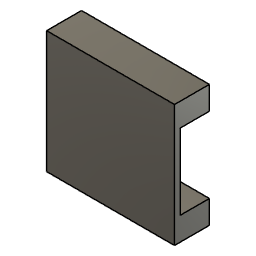
磁铁测试底座 (Autodesk Fusion 360 design; units mm, degrees)
Autodesk Fusion 360 part; units mm, degrees
note: some values were not read from the file. Chosen so that the rebuilt part matches the saved one: which bodies a step acts on.
sketch "草图1" plane through (0, 0, 0) normal (0, 1, 0) x (1, 0, 0)
  line L0 (0, 0) -> (22, 0)
  line L1 (22, 0) -> (22, -6)
  line L2 (22, -6) -> (0, -6)
  line L3 (0, -6) -> (0, 0)
  line L4 (1, -5) -> (21, -5)
  line L5 (21, -5) -> (21, 0)
  line L6 (21, 0) -> (1, 0)
  line L7 (1, 0) -> (1, -5)
  dimension "d1" = 22
  dimension "d2" = 6
  dimension "d3" = 1
  dimension "d4" = 1
  dimension "d5" = 1
  constraint horizontal L0
  constraint vertical L1
  constraint horizontal L2
  constraint vertical L3
  constraint coincident L0.start L3.end
  constraint horizontal L4
  constraint vertical L5
  constraint horizontal L6
  constraint vertical L7
  constraint coincident L0 L5.end
  measures "d1" distance of L0.start L0.end
  measures "d2" distance of L0.start L2.end
  measures "d3" distance of L2 L4
  measures "d4" distance of L3 L7
  measures "d5" distance of L1 L5
extrude "拉伸1" add sketch "草图1" along normal blind 21 contours L0 L1 L2 L3 L4 L5 L7 makes body 1
extrude "拉伸2" add sketch "草图1" along normal blind 1 separate body contours L0 L4 L5 L6 L7 makes body 2
sketch "草图2" plane through (0, 0, 5) normal (0, 0, -1) x (-1, 0, 0)
  line L0 (-21, 0) -> (-1, 0)
  line L1 (-1, 0) -> (-1, 21)
  line L2 (-1, 21) -> (-21, 21)
  line L3 (-21, 21) -> (-21, 0)
  line L4 (-1, 20) -> (-21, 20)
  line L5 (-21, 20) -> (-21, 21)
  line L6 (-21, 21) -> (-1, 21)
  line L7 (-1, 21) -> (-1, 20)
  line L8 (-21, 20) -> (-21, 18)
  line L9 (-1, 1) -> (-1, 3)
  line L10 (-22, 18) -> (0, 18)
  line L11 (0, 18) -> (0, 3)
  line L12 (0, 3) -> (-22, 3)
  line L13 (-22, 3) -> (-22, 18)
  dimension "d10" = 1
  constraint horizontal L4
  constraint vertical L5
  constraint horizontal L6
  constraint vertical L7
  constraint coincident L2.end L3.start
  constraint coincident L1 L4.start
  constraint coincident L3 L8.end
  constraint perpendicular L4 L8
  constraint coincident L1 L9.start
  constraint coincident L1 L9.end
  constraint horizontal L10
  constraint vertical L11
  constraint horizontal L12
  constraint vertical L13
  measures "d10" distance of L4 L6
extrude "拉伸3" add sketch "草图2" along normal blind 5 contours L1 L2 L3 L4 L5 L6 L7 bodies 1
sketch "草图3" plane through (0, 0, 5) normal (0, 0, -1) x (-1, 0, 0)
  line L0 (-1, 20) -> (-21, 20)
  line L1 (-21, 20) -> (-21, 0)
  line L2 (-21, 0) -> (-1, 0)
  line L3 (-1, 0) -> (-1, 20)
  line L4 (-1, 1) -> (-1, 3)
  line L5 (-1, 20) -> (-1, 18)
  line L6 (-1, 3) -> (0, 3)
  line L7 (0, 3) -> (0, 18)
  line L8 (0, 18) -> (-1, 18)
  line L9 (-1, 18) -> (-1, 3)
  line L10 (-21, 3) -> (-22, 3)
  line L11 (-22, 3) -> (-22, 18)
  line L12 (-22, 18) -> (-21, 18)
  line L13 (-21, 18) -> (-21, 3)
  line L14 (0, 10.5) -> (-11, 10.5) construction
  line L15 (-11, 10.5) -> (-11, 10) construction
  line L16 (-11, 10) -> (-15, 10)
  line L17 (-15, 10) -> (-17.5, 9.5)
  line L18 (-17.5, 9.5) -> (-15, 9)
  line L19 (-15, 9) -> (-7.5, 9)
  line L20 (-7.5, 9) -> (-5, 9.5)
  line L21 (-5, 9.5) -> (-7.5, 10)
  line L22 (-7.5, 10) -> (-11, 10)
  line L23 (-22, 10) -> (0, 10)
  dimension "d13" = 2
  dimension "d14" = 2
  constraint coincident L3 L4.start
  constraint coincident L0.start L3.end
  constraint coincident L3 L5.end
  constraint horizontal L6
  constraint vertical L7
  constraint horizontal L8
  constraint vertical L9
  constraint horizontal L10
  constraint vertical L11
  constraint horizontal L12
  constraint vertical L13
  constraint coincident L1 L10.start
  constraint midpoint L7 L14.start
  constraint perpendicular L11 L14
  constraint perpendicular L14 L15
  constraint perpendicular L15 L16
  constraint parallel L16 L19
  constraint parallel L17 L20
  constraint parallel L18 L21
  constraint perpendicular L15 L22
  constraint coincident L11 L23.start
  constraint coincident L7 L23.end
  constraint perpendicular L7 L23
  measures "d13" distance of L4.start L4.end
  measures "d14" distance of L0.start L5.end
extrude "拉伸5" cut sketch "草图3" against normal blind 1 contours L16 L17 L18 L19 L20 L21 L22 L23 bodies 1
pattern_linear "R-阵列1" count 9 spacing 1 along (0, -1, 0) of "拉伸5"
extrude "拉伸1'" add sketch "草图3" against normal blind 1 separate body contours L16 L17 L18 L19 L20 L21 L22 L23 makes body 3 in component "Component'"
pattern_linear "R-阵列1'" count 9 spacing 1 along (0, -1, 0) of "拉伸1'" makes body 4 makes body 5 makes body 6 makes body 7 makes body 8 makes body 9 makes body 10 makes body 11 in component "Component'"
split "分割1" by curves path "草图3" along L23 bodies 1 makes body 12 at (1.6667, 4.8333, 6)
sketch "草图4" plane through (0, 0, 6) normal (0, 0, 1) x (1, 0, 0)
  line L0 (22, 10) -> (15, 10)
  line L1 (15, 10) -> (17.5, 9.5)
  line L2 (17.5, 9.5) -> (15, 9)
  line L3 (15, 9) -> (17.5, 8.5)
  line L4 (17.5, 8.5) -> (15, 8)
  line L5 (15, 8) -> (17.5, 7.5)
  line L6 (17.5, 7.5) -> (15, 7)
  line L7 (15, 7) -> (17.5, 6.5)
  line L8 (17.5, 6.5) -> (15, 6)
  line L9 (15, 6) -> (17.5, 5.5)
  line L10 (17.5, 5.5) -> (15, 5)
  line L11 (15, 5) -> (17.5, 4.5)
  line L12 (17.5, 4.5) -> (15, 4)
  line L13 (15, 4) -> (17.5, 3.5)
  line L14 (17.5, 3.5) -> (15, 3)
  line L15 (15, 3) -> (17.5, 2.5)
  line L16 (17.5, 2.5) -> (15, 2)
  line L17 (15, 2) -> (17.5, 1.5)
  line L18 (17.5, 1.5) -> (15, 1)
  line L19 (15, 1) -> (7.5, 1)
  line L20 (7.5, 1) -> (5, 1.5)
  line L21 (5, 1.5) -> (7.5, 2)
  line L22 (7.5, 2) -> (5, 2.5)
  line L23 (5, 2.5) -> (7.5, 3)
  line L24 (7.5, 3) -> (5, 3.5)
  line L25 (5, 3.5) -> (7.5, 4)
  line L26 (7.5, 4) -> (5, 4.5)
  line L27 (5, 4.5) -> (7.5, 5)
  line L28 (7.5, 5) -> (5, 5.5)
  line L29 (5, 5.5) -> (7.5, 6)
  line L30 (7.5, 6) -> (5, 6.5)
  line L31 (5, 6.5) -> (7.5, 7)
  line L32 (7.5, 7) -> (5, 7.5)
  line L33 (5, 7.5) -> (7.5, 8)
  line L34 (7.5, 8) -> (5, 8.5)
  line L35 (5, 8.5) -> (7.5, 9)
  line L36 (7.5, 9) -> (5, 9.5)
  line L37 (5, 9.5) -> (7.5, 10)
  line L38 (7.5, 10) -> (0, 10)
  line L39 (0, 10) -> (0, 0)
  line L40 (0, 0) -> (22, 0)
  line L41 (22, 0) -> (22, 10)
  line L42 (7.5, 1) -> (15, 1)
  line L43 (15, 1) -> (15, 0)
  line L44 (15, 0) -> (7.5, 0)
  line L45 (7.5, 0) -> (7.5, 1)
  constraint horizontal L42
  constraint vertical L43
  constraint horizontal L44
  constraint vertical L45
  constraint coincident L40 L43.end
  constraint coincident L19.end L20.start
split "分割2" by curves path "草图4" along L45 L42 L43 L44 bodies 12 makes body 13 at (1.6667, 4.8333, 6) makes body 14 at (22, 3.3333, 2)
combine "合并1" operation add target body 12 tool bodies 2
combine "合并2" operation add target body 13 tool bodies 14 1
extrude "拉伸6" add sketch "草图3" against normal blind 1 separate body contours L16 L17 L18 L19 L20 L21 L22 L23 makes body 15
pattern_linear "R-阵列2" count 9 spacing 1 along (0, -1, 0) of "拉伸6" makes body 16 makes body 17 makes body 18 makes body 19 makes body 20 makes body 21 makes body 22 makes body 23
combine "合并3" operation add target body 23 tool bodies 16 21 17 15 18 19 20 22
combine "合并4" operation add target body 12 tool bodies 23
sketch "草图5" plane through (0, 0, 0) normal (0, 0, -1) x (-1, 0, 0)
  line L0 (-1, 20) -> (-1, 0)
  line L1 (-1, 0) -> (0, 0)
  line L2 (0, 0) -> (0, 21)
  line L3 (0, 21) -> (-22, 21)
  line L4 (-22, 21) -> (-22, 0)
  line L5 (-22, 0) -> (-21, 0)
  line L6 (-21, 0) -> (-21, 20)
  line L7 (-21, 20) -> (-1, 20)
  line L8 (-21, 1) -> (-21, 3)
  line L9 (-21, 0) -> (-22, 0)
  line L10 (-22, 0) -> (-22, 3)
  line L11 (-22, 3) -> (-21, 3)
  line L12 (-21, 3) -> (-21, 0)
  line L13 (0, 0) -> (-1, 0)
  line L14 (-1, 0) -> (-1, 3)
  line L15 (-1, 3) -> (0, 3)
  line L16 (0, 3) -> (0, 0)
  constraint coincident L6 L8.start
  constraint coincident L6 L8.end
  constraint horizontal L9
  constraint vertical L10
  constraint horizontal L11
  constraint vertical L12
  constraint coincident L4 L10.end
  constraint coincident L5.end L6.start
  constraint horizontal L13
  constraint vertical L14
  constraint horizontal L15
  constraint vertical L16
  constraint coincident L0 L14.end
  constraint coincident L1.end L2.start
split "分割3" by curves path "草图5" along L12 L9 L10 L11 bodies 13 makes body 24 at (9.8333, 17.3333, 6)
split "分割4" by curves path "草图5" along L16 L13 L14 L15 bodies 24 makes body 25 at (9.8333, 17.3333, 6)
combine "合并5" operation add target body 24 tool bodies 13 12
extrude "拉伸7" cut sketch "草图2" along normal blind 5 contours L3 L10 L12 L13 | L1 L10 L11 L12 bodies 25
combine "合并6" operation add target body 25 tool bodies 24
sketch "草图6" plane through (0, 0, 5) normal (0, 0, -1) x (-1, 0, 0)
  line L0 (-21, 1) -> (-1, 1)
  line L1 (-1, 1) -> (-1, 3)
  line L2 (-1, 3) -> (0, 3)
  line L3 (0, 3) -> (0, 18)
  line L4 (0, 18) -> (-1, 18)
  line L5 (-1, 18) -> (-1, 20)
  line L6 (-1, 20) -> (-21, 20)
  line L7 (-21, 20) -> (-21, 18)
  line L8 (-21, 18) -> (-22, 18)
  line L9 (-22, 18) -> (-22, 3)
  line L10 (-22, 3) -> (-21, 3)
  line L11 (-21, 3) -> (-21, 1)
  line L12 (-21.5, 3) -> (-21, 3)
  line L13 (-0.5, 3) -> (-1, 3)
  line L14 (0, 4) -> (-22, 4)
  line L15 (-22, 4) -> (-22, 3.2)
  line L16 (-22, 3.2) -> (0, 3.2)
  line L17 (0, 3.2) -> (0, 4)
  line L18 (0, 17) -> (-22, 17)
  line L19 (-22, 17) -> (-22, 17.8)
  line L20 (-22, 17.8) -> (0, 17.8)
  line L21 (0, 17.8) -> (0, 17)
  line L22 (-1, 1) -> (-0.75, 1)
  line L23 (-0.75, 1) -> (-0.75, 3)
  line L24 (-0.75, 3) -> (-1, 3)
  line L25 (-1, 3) -> (-1, 1)
  line L26 (-21, 1) -> (-21.25, 1)
  line L27 (-21.25, 1) -> (-21.25, 3)
  line L28 (-21.25, 3) -> (-21, 3)
  line L29 (-21, 3) -> (-21, 1)
  line L30 (-21, 20) -> (-21.25, 20)
  line L31 (-21.25, 20) -> (-21.25, 18)
  line L32 (-21.25, 18) -> (-21, 18)
  line L33 (-21, 18) -> (-21, 20)
  line L34 (-1, 20) -> (-0.75, 20)
  line L35 (-0.75, 20) -> (-0.75, 18)
  line L36 (-0.75, 18) -> (-1, 18)
  line L37 (-1, 18) -> (-1, 20)
  line L38 (-22, 18) -> (-21, 18)
  line L39 (-21, 18) -> (-21, 17.8)
  line L40 (-21, 17.8) -> (-22, 17.8)
  line L41 (-22, 17.8) -> (-22, 18)
  line L42 (-22, 3.2) -> (-21, 3.2)
  line L43 (-21, 3.2) -> (-21, 3)
  line L44 (-21, 3) -> (-22, 3)
  line L45 (-22, 3) -> (-22, 3.2)
  line L46 (0, 3.2) -> (-1, 3.2)
  line L47 (-1, 3.2) -> (-1, 3)
  line L48 (-1, 3) -> (0, 3)
  line L49 (0, 3) -> (0, 3.2)
  line L50 (-1, 18.2125) -> (0, 18.2125)
  line L51 (0, 18.2125) -> (0, 18)
  line L52 (0, 18) -> (-1, 18)
  line L53 (-1, 18) -> (-1, 18.2125)
  line L54 (-1, 18) -> (0, 18)
  line L55 (0, 18) -> (0, 17.8)
  line L56 (0, 17.8) -> (-1, 17.8)
  line L57 (-1, 17.8) -> (-1, 18)
  dimension "d39" = 0.8
  dimension "d40" = 0.8
  dimension "d43" = 0.25
  dimension "d44" = 0.25
  dimension "d45" = 0.25
  dimension "d46" = 0.25
  constraint horizontal L12
  constraint horizontal L13
  constraint midpoint L2 L13.start
  constraint horizontal L14
  constraint vertical L15
  constraint horizontal L16
  constraint vertical L17
  constraint coincident L3 L14.start
  constraint horizontal L18
  constraint vertical L19
  constraint horizontal L20
  constraint vertical L21
  constraint coincident L3 L18.start
  constraint horizontal L22
  constraint vertical L23
  constraint horizontal L24
  constraint vertical L25
  constraint coincident L0.end L1.start
  constraint horizontal L26
  constraint vertical L27
  constraint horizontal L28
  constraint vertical L29
  constraint coincident L0.start L11.end
  constraint horizontal L30
  constraint vertical L31
  constraint horizontal L32
  constraint vertical L33
  constraint coincident L6.end L7.start
  constraint horizontal L34
  constraint vertical L35
  constraint horizontal L36
  constraint vertical L37
  constraint coincident L5.end L6.start
  constraint horizontal L38
  constraint vertical L39
  constraint horizontal L40
  constraint vertical L41
  constraint coincident L20 L39.end
  constraint coincident L8.end L9.start
  constraint horizontal L42
  constraint vertical L43
  constraint horizontal L44
  constraint vertical L45
  constraint horizontal L46
  constraint vertical L47
  constraint horizontal L48
  constraint vertical L49
  constraint coincident L1.end L2.start
  constraint horizontal L50
  constraint vertical L51
  constraint horizontal L52
  constraint vertical L53
  constraint coincident L3.end L4.start
  constraint coincident L37 L50.start
  constraint horizontal L54
  constraint vertical L55
  constraint horizontal L56
  constraint vertical L57
  constraint coincident L4.end L5.start
  measures "d39" distance of L14.start L16.end
  measures "d40" distance of L18.start L20.end
  measures "d43" distance of L0.end L22.end
  measures "d44" distance of L0.start L26.end
  measures "d45" distance of L6.end L30.end
  measures "d46" distance of L5.end L34.end
extrude "拉伸10" cut sketch "草图6" along normal blind 5 contours L10 L11 L12 L26 L27 L28 L29 L44 | L1 L2 L13 L22 L23 L24 L25 L48 | L7 L8 L30 L31 L32 L33 L38 | L4 L5 L35 L36 L37 L50 L52 L53 L54 | L5 L34 L35 L37 L50 bodies 25
extrude "拉伸11" add sketch "草图6" along normal blind 5 contours L9 L10 L12 L16 L28 L42 L43 L44 L45 | L2 L3 L13 L16 L24 L46 L47 L48 L49 | L8 L9 L20 L32 L38 L39 L40 L41 | L3 L4 L20 L36 L52 L54 L55 L56 L57 bodies 25
extrude "拉伸12" add sketch "草图6" along normal blind 5 contours L3 L9 L14 L15 L16 L17 L42 L46 | L3 L9 L18 L19 L20 L21 L40 L56 bodies 25
sketch "草图7" plane through (0, 0, 0) normal (0, 0, -1) x (-1, 0, 0)
  line L0 (-22, 4) -> (-22, 0)
  line L1 (-22, 0) -> (0, 0)
  line L2 (0, 0) -> (0, 4)
  line L3 (0, 4) -> (-22, 4)
  line L4 (-21, 3.2) -> (-1, 3.2)
  line L5 (-1, 3.2) -> (-1, 3)
  line L6 (-1, 3) -> (-0.75, 3)
  line L7 (-0.75, 3) -> (-0.75, 1)
  line L8 (-0.75, 1) -> (-21.25, 1)
  line L9 (-21.25, 1) -> (-21.25, 3)
  line L10 (-21.25, 3) -> (-21, 3)
  line L11 (-21, 3) -> (-21, 3.2)
  line L12 (-21, 3.2) -> (-1, 3.2)
  line L13 (-1, 3.2) -> (-1, 3)
  line L14 (-1, 3) -> (-21, 3)
  line L15 (-21, 3) -> (-21, 3.2)
  line L16 (-1, 18) -> (-21, 18)
  line L17 (-21, 18) -> (-21, 17.8)
  line L18 (-21, 17.8) -> (-1, 17.8)
  line L19 (-1, 17.8) -> (-1, 18)
  constraint horizontal L12
  constraint vertical L13
  constraint horizontal L14
  constraint vertical L15
  constraint coincident L5.end L6.start
  constraint coincident L4.start L11.end
  constraint horizontal L16
  constraint vertical L17
  constraint horizontal L18
  constraint vertical L19
extrude "拉伸13" add sketch "草图7" against normal blind 0.2 contours L4 L5 L11 L12 L13 L14 L15 | L16 L17 L18 L19 bodies 25
component "Component'" placed x (1, 0, 0) y (0, 1, 0) z (0, 0, 1) at (0, 0, 0)
